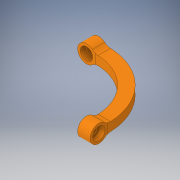
# Autodesk Inventor part: Link
Saved by Autodesk Inventor 2019 (Build 230136000, 136)
## iProperties
Created: 2022-07-05
Part Number: Link
Material: Generic
Document SubType Name: Modeling
Designer: zreik
Density: 1 g/cm^3
Appearance: Orange
Author: zreik
Autodesk Inventor part; units mm, degrees
ref_plane "XZ Plane" through (0, 0, 0) normal (0, 1, 0) x (-1, 0, 0)
ref_plane "XY Plane" through (0, 0, 0) normal (0, 0, 1) x (1, 0, 0)
sketch "Sketch1" plane through (0, 0, 0) normal (0, 0, 1) x (1, 0, 0)
  circle A0 centre (0, 0) radius 5
  dimension "d0" = 10
  constraints: 1 centre point, 1 coincident
  measures "d0" diameter of A0
extrude "Extrusion1" add sketch "Sketch1" along normal blind 7
sketch "Sketch2" plane through (0, 0, 0) normal (1, 0, 0) x (0, 1, 0)
  line L0 (-2.5, 7) -> (2.5, 7)
  line L1 (2.5, 7) -> (2.5, 0)
  line L2 (2.5, 0) -> (-2.5, 0)
  line L3 (-2.5, 0) -> (-2.5, 7)
  line L4 (-2.5, 7) -> (2.5, 0) construction
  line L5 (2.5, 7) -> (-2.5, 0) construction
  line L6 (-5, 0) -> (5, 0) projected
  point P0 (0, 0)
  point P1 (0, 3.5)
  dimension "d3" = 3.5
  dimension "d4" = 0
  dimension "d5" = 7
  dimension "d6" = 5
  constraints: 12 end point, 2 midpoint, 2 parallel, 1 horizontal, 1 perpendicular
  measures "d3" distance from line of L6 point (0, 3.5)
  measures "d4" horizontal distance of point (0, 0) point (0, 3.5)
  measures "d5" distance of L0.end L1.end
  measures "d6" distance of L1.end L2.end
sketch "Sketch3" plane through (0, 0, 0) normal (0, 1, 0) x (-1, 0, 0)
  arc A0 (-40, 37.5) -> (-5, 2.5) centre (-5, 37.5) ccw
  line L0 (-5, 2.5) -> (0, 2.5)
  line L1 (-40, 37.5) -> (-40, 42.5)
  point P0 (0, 0)
  dimension "d14" = 2.5
  dimension "d15" = 5
  dimension "d17" = 5
  dimension "d24" = 5
  dimension "d55" = 35
  dimension "d56" = 0
  dimension "d57" = 35
  constraints: 4 end point, 2 point on circle, 1 centre point, 1 horizontal, 1 vertical
  measures "d14" vertical distance of point (0, 0) L0.start
  measures "d15" horizontal distance of L0.start point (0, 0)
  measures "d17" distance of L0.start L0.end
  measures "d24" distance of L1.start L1.end
  measures "d55" horizontal distance of L0.start L1.start
  measures "d56" vertical distance of L1.start A0.centre
  measures "d57" horizontal distance of L0.start L1.start
sweep "Sweep1" add profiles "Sketch2" path "Sketch3" path curves L0 A0 L1
ref_plane "Work Plane1" through (39, 0, 0) normal (1, 0, 0) x (0, 1, 0)
sketch "Sketch4" plane through (39, 0, 0) normal (1, 0, 0) x (0, 1, 0)
  circle A0 centre (0, 42.5) radius 5
  point P0 (0, 0)
  dimension "d27" = 10
  dimension "d28" = 42.5
  dimension "d29" = 0
  constraints: 1 centre point
  measures "d27" diameter of A0
  measures "d28" distance of A0.centre point (0, 0)
  measures "d29" horizontal distance of point (0, 0) A0.centre
extrude "Extrusion2" add sketch "Sketch4" along normal mid plane 7
sketch "Sketch6" plane through (42.5, -2.5, 37.5) normal (-1, 0, 0) x (0, 0, 1)
  circle A0 centre (5, 2.5) radius 3.5
  point P0 (-37.5, 2.5)
  dimension "d32" = 7
  dimension "d33" = 42.5
  dimension "d34" = 0
  constraints: 1 centre point
  measures "d32" diameter of A0
  measures "d33" distance of point (-37.5, 2.5) A0.centre
  measures "d34" vertical distance of A0.centre point (-37.5, 2.5)
extrude "Extrusion4" cut sketch "Sketch6" along normal blind 3
sketch "Sketch7" plane through (39.5, 0, 42.5) normal (-1, 0, 0) x (0, 0, 1)
  circle A0 centre (0, 0) radius 2.5
  line L0 (-42.5, 5) -> (-42.5, -5) projected
  point P0 (-42.5, 0)
  point P1 (-42.5, -2.5)
  point P2 (-42.5, 2.5)
  dimension "d37" = 5
  dimension "d38" = 42.5
  dimension "d39" = 0
  constraints: 1 centre point
  measures "d37" diameter of A0
  measures "d38" distance from line of A0.centre L0
  measures "d39" vertical distance of point (-42.5, 0) A0.centre
extrude "Extrusion5" cut sketch "Sketch7" along normal up to next
sketch "Sketch8" plane through (0, 0, 0) normal (0, 0, -1) x (-1, 0, 0)
  circle A0 centre (0, 0) radius 3.5
  dimension "d42" = 7
  constraints: 1 centre point, 1 coincident
  measures "d42" diameter of A0
extrude "Extrusion6" cut sketch "Sketch8" against normal blind 3
sketch "Sketch9" plane through (0, 0, 3) normal (0, 0, -1) x (-1, 0, 0)
  circle A0 centre (0, 0) radius 2.5
  dimension "d45" = 5
  constraints: 1 centre point, 1 coincident
  measures "d45" diameter of A0
extrude "Extrusion7" cut sketch "Sketch9" against normal up to next
fillet "Fillet1" radius 5 4 edges at (39, -2.5, 38.1699) (4.3301, -2.5, 3.5) (4.3301, 2.5, 3.5) (39, 2.5, 38.1699)
sketch "Sketch10" plane through (35.5, 0, 42.5) normal (-1, 0, 0) x (0, 0, 1)
  circle A0 centre (0, 0) radius 3.5
  circle A1 centre (0, 0) radius 2.5 projected
  point P0 (-42.5, 0)
  dimension "d49" = 7
  constraints: 1 centre point, 1 concentric
  measures "d49" diameter of A0
extrude "Extrusion8" cut sketch "Sketch10" against normal blind 3
sketch "Sketch11" plane through (0, 0, 7) normal (0, 0, 1) x (1, 0, 0)
  circle A0 centre (0, 0) radius 3.5
  circle A1 centre (0, 0) radius 2.5 projected
  dimension "d52" = 7
  constraints: 1 centre point, 1 concentric
  measures "d52" diameter of A0
extrude "Extrusion9" cut sketch "Sketch11" against normal blind 3
equation "\"d3\" = 0.5 * d5"
equation "\"d55\" = width"
equation "\"d57\" = height"
equation "\"d33\" = d28"
equation "\"d38\" = d28"
equation "\"width\" = 35"
equation "\"height\" = 35"
body "Solid1"
